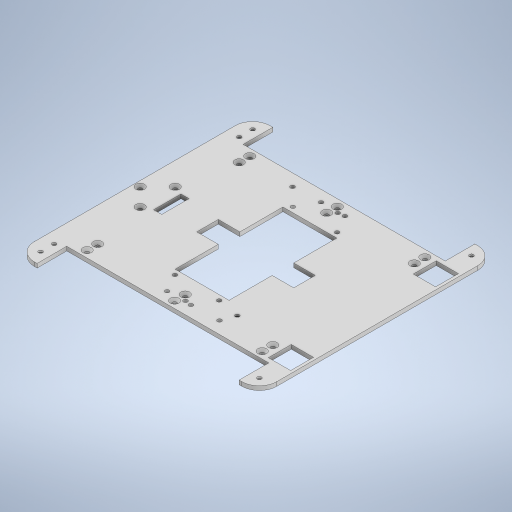
# Autodesk Inventor part: base
Saved by Autodesk Inventor 2023 (Build 270158000, 158)
## iProperties
Created: 2026-02-09
Part Number: base
Material: Типовые
Document SubType Name: Modeling
Designer: garin
Density: 1 g/cm^3
Appearance: По умолчанию
Author: garin
Autodesk Inventor part; units mm, degrees
ref_plane "YZ Plane" through (0, 0, 0) normal (1, 0, 0) x (0, 1, 0)
ref_plane "XZ Plane" through (0, 0, 0) normal (0, 1, 0) x (-1, 0, 0)
ref_plane "XY Plane" through (0, 0, 0) normal (0, 0, 1) x (1, 0, 0)
sketch "Эскиз1" plane through (0, 0, 0) normal (0, 1, 0) x (-1, 0, 0)
  line L0 (-77, -87.5) -> (77, -87.5)
  line L1 (90, -74.5) -> (90, 74.5)
  line L2 (77, 87.5) -> (-77, 87.5)
  line L3 (-90, 74.5) -> (-90, -74.5)
  line L4 (90, 0) -> (-90, 0) construction
  line L5 (0, -87.5) -> (0, 87.5) construction
  arc A0 (90, 74.5) -> (77, 87.5) centre (77, 74.5) ccw
  arc A1 (77, -87.5) -> (90, -74.5) centre (77, -74.5) ccw
  arc A2 (-90, -74.5) -> (-77, -87.5) centre (-77, -74.5) ccw
  arc A3 (-77, 87.5) -> (-90, 74.5) centre (-77, 74.5) ccw
  line L6 (75, 83.5) -> (-75, 83.5)
  line L7 (-75, 83.5) -> (-75, 65.5)
  line L8 (-75, 65.5) -> (75, 65.5)
  line L9 (75, 65.5) -> (75, 83.5)
  line L10 (0, 87.5) -> (0, -87.5) construction
  line L11 (75, -83.5) -> (-75, -83.5)
  line L12 (-75, -83.5) -> (-75, -65.5)
  line L13 (-75, -65.5) -> (75, -65.5)
  line L14 (75, -65.5) -> (75, -83.5)
  line L15 (90, 49.8397) -> (90, 20.3597)
  line L16 (0, 65.5) -> (42, 65.5)
  line L17 (90, -32.9125) -> (90, 38.6688)
  line L18 (68, 60) -> (-12, 60)
  line L19 (-12, 60) -> (-12, -60)
  line L20 (-12, -60) -> (68, -60)
  line L21 (68, -60) -> (68, 60)
  line L22 (60, 60) -> (57.2, 60)
  line L23 (60, 57.2) -> (60, 60)
  circle A4 centre (65.2, 57.2) radius 1.5
  line L24 (20, 60) -> (20, -60) construction
  circle A5 centre (65.2, -57.2) radius 1.5
  circle A6 centre (-9.2, 57.2) radius 1.5
  circle A7 centre (-9.2, -57.2) radius 1.5
  line L25 (-20, 0) -> (-25, 0) construction
  line L26 (-25, 0) -> (-81, 0) construction
  line L27 (-13, 42.5) -> (-69, 42.5)
  line L28 (-69, 42.5) -> (-69, -42.5)
  line L29 (-69, -42.5) -> (-13, -42.5)
  line L30 (-13, -42.5) -> (-13, 42.5)
  line L31 (-25, 42.5) -> (-28.7, 42.5)
  line L32 (-25, 38.8) -> (-25, 42.5)
  circle A8 centre (-16.7, 38.8) radius 1.5
  line L33 (-53, 42.5) -> (-53, -42.5) construction
  line L34 (-25, 0) -> (-81, 0) construction
  line L35 (-16.7, 38.8) -> (-16.7, -19.2) construction
  circle A9 centre (-16.7, -19.2) radius 1.5
  circle A10 centre (-65.3, 38.8) radius 1.5
  circle A11 centre (-65.3, -19.2) radius 1.5
  line L36 (90, 60.5) -> (90, 65.5)
  circle A12 centre (65, 60.3847) radius 1.5
  circle A13 centre (65, 52.5) radius 1.5
  line L37 (32.5, 60.3847) -> (32.5, -60) construction
  circle A14 centre (0, 60.3847) radius 1.5
  circle A15 centre (0, 52.5) radius 1.5
  circle A16 centre (-65, 60.3847) radius 1.5
  circle A17 centre (-65, 52.5) radius 1.5
  circle A18 centre (65, -60.3847) radius 1.5
  circle A19 centre (65, -52.5) radius 1.5
  circle A20 centre (0, -60.3847) radius 1.5
  circle A21 centre (0, -52.5) radius 1.5
  circle A22 centre (-65, -60.3847) radius 1.5
  circle A23 centre (-65, -52.5) radius 1.5
  circle A24 centre (86, 0) radius 1.5
  line L38 (86, 0) -> (104.385, 0) construction
  circle A25 centre (72.9998, -13.0002) radius 1.5
  circle A26 centre (72.9998, 12.9998) radius 1.5
  line L39 (90, -19.2) -> (75, -19.2)
  line L40 (75, -19.2) -> (75, 22.1472)
  line L41 (75, 22.1472) -> (90, 22.1472)
  line L42 (90, 22.1472) -> (90, -19.2)
  line L43 (-90, 8.1057) -> (-90, 0)
  line L44 (0, 0) -> (-12, 0)
  line L45 (-12, 5.1924) -> (-12, 5.1924)
  line L46 (75, 78.692) -> (75, 65.5)
  circle A27 centre (81.192, 78.692) radius 1.5
  circle A28 centre (81.192, -78.692) radius 1.5
  circle A29 centre (81.192, 68.692) radius 1.5
  circle A30 centre (81.192, -68.692) radius 1.5
  line L47 (66.2, 9.8) -> (66.2, -10.5)
  line L48 (66.2, -10.5) -> (60.2, -10.5)
  line L49 (60.2, -10.5) -> (60.2, 9.8)
  line L50 (60.2, 9.8) -> (66.2, 9.8)
  circle A31 centre (-81.192, -78.692) radius 1.5
  circle A32 centre (-81.192, 78.692) radius 1.5
  line L51 (0, 0) -> (-71.5, 0) construction
  line L52 (-71.5, 0) -> (-71.5, 45.306) construction
  line L53 (-71.5, 45.306) -> (0, 45.306) construction
  line L54 (0, 45.306) -> (0, 0) construction
  line L55 (-71.5, 45.306) -> (-88, 45.306)
  line L56 (-88, 45.306) -> (-88, 62.3062)
  line L57 (-88, 62.3062) -> (-71.5, 62.3062)
  line L58 (-71.5, 62.3062) -> (-71.5, 45.306)
  line L59 (-71.5, -45.306) -> (-88, -45.306)
  line L60 (-88, -45.306) -> (-88, -62.3062)
  line L61 (-88, -62.3062) -> (-71.5, -62.3062)
  line L62 (-71.5, -62.3062) -> (-71.5, -45.306)
  line L63 (20, -40) -> (-20, -40)
  line L64 (-20, -40) -> (-20, 40)
  line L65 (-20, 40) -> (20, 40)
  line L66 (20, 40) -> (20, -40)
  line L67 (20, 0) -> (-20, 0) construction
  line L68 (0, -40) -> (0, 40) construction
  line L69 (0, 65.5) -> (-4.2, 65.5) construction
  line L70 (-4.2, 65.5) -> (-4.2, 56.5) construction
  line L71 (-4.2, 56.5) -> (0, 56.5) construction
  line L72 (0, 56.5) -> (0, 65.5) construction
  circle A33 centre (-4.2, 56.5) radius 1.5
  line L73 (0, 65.5) -> (-29.4, 65.5) construction
  line L74 (-29.4, 65.5) -> (-29.4, 56.5) construction
  line L75 (-29.4, 56.5) -> (0, 56.5) construction
  line L76 (0, 56.5) -> (0, 65.5) construction
  circle A34 centre (-29.4, 56.5) radius 1.5
  circle A35 centre (-4.2, -56.5) radius 1.5
  circle A36 centre (29.4, -56.5) radius 1.5
  line L77 (0, 60.3847) -> (8.833, 60.3847)
  line L78 (8.833, 60.3847) -> (8.833, 57.162)
  line L79 (8.833, 57.162) -> (0, 57.162)
  line L80 (0, 57.162) -> (0, 60.3847)
  circle A37 centre (8.833, 57.162) radius 1.5
  circle A38 centre (-8.833, 57.162) radius 1.5
  circle A39 centre (8.833, -57.162) radius 1.5
  circle A40 centre (-8.833, -57.162) radius 1.5
  line L81 (-20, 0) -> (-20, -8)
  line L82 (-20, -8) -> (-36, -8)
  line L83 (-36, -8) -> (-36, 8)
  line L84 (-36, 8) -> (-20, 8)
  line L85 (-20, 8) -> (-20, -8)
  line L86 (20, -8) -> (36, -8)
  line L87 (36, -8) -> (36, 8)
  line L88 (36, 8) -> (20, 8)
  line L89 (20, 8) -> (20, -8)
  line L90 (0, 0) -> (16.43, 0) construction
  line L91 (16.43, 0) -> (16.43, 43.8) construction
  line L92 (16.43, 43.8) -> (0, 43.8) construction
  line L93 (0, 43.8) -> (0, 0) construction
  circle A41 centre (16.43, 43.8) radius 1.5
  circle A42 centre (-16.43, 43.8) radius 1.5
  circle A43 centre (16.43, -43.8) radius 1.5
  circle A44 centre (-16.43, -43.8) radius 1.5
  line L94 (0, 0) -> (-32.9, 0) construction
  line L95 (-32.9, 0) -> (-32.9, 46.85) construction
  line L96 (-32.9, 46.85) -> (0, 46.85) construction
  line L97 (0, 46.85) -> (0, 0) construction
  circle A45 centre (-32.9, 46.85) radius 1.5
  line L98 (0, -83.5) -> (3, -83.5)
  line L99 (3, -83.5) -> (-3, -83.5)
  line L100 (-3, -83.5) -> (-3, -65.5)
  line L101 (-3, -65.5) -> (3, -65.5)
  line L102 (3, -65.5) -> (3, -83.5)
  line L103 (-3, 83.5) -> (-3, 65.5)
  line L104 (3, 65.5) -> (3, 83.5)
  line L105 (75, 83.5) -> (75, 87.5)
  line L106 (-75, 83.5) -> (-75, 87.5)
  line L107 (75, -83.5) -> (75, -87.5)
  line L108 (-75, -83.5) -> (-75, -87.5)
  point P0 (90, 87.5)
  point P1 (90, -87.5)
  point P2 (-90, 87.5)
  point P3 (-77, -74.5)
  point P4 (60, 0)
  point P5 (75, 0)
  point P6 (60, 0)
  point P7 (-60, 0)
  point P8 (-4, 0)
  point P9 (-5, 0)
  point P10 (-15, 0)
  point P11 (-70, 0)
  point P12 (-14, 0)
  point P13 (-28.7, -19.2)
  point P14 (-17.7, -19.2)
  point P15 (-13, 0)
  point P16 (-14, 0)
  point P17 (-17.6, 40)
  point P18 (-15.8, 40)
  dimension "d0" = 180
  dimension "d1" = 175
  dimension "d2" = 13
  dimension "d7" = 150
  dimension "d8" = 18
  dimension "d13" = 80
  dimension "d14" = 120
  dimension "d21" = 56
  dimension "d22" = 85
  dimension "d25" = 3
  dimension "d26" = 58
  dimension "d27" = 3
  dimension "d30" = 3
  dimension "d32" = 3
  dimension "d33" = 32.5
  dimension "d54" = 3
  dimension "d58" = 3
  dimension "d59" = 3
  dimension "d60" = 15
  dimension "d62" = 12
  dimension "d68" = 3
  dimension "d70" = 3
  dimension "d72" = 20.3
  dimension "d73" = 6
  dimension "d76" = 3
  dimension "d77" = 71.5
  dimension "d78" = 45.306
  dimension "d79" = 40
  dimension "d80" = 80
  dimension "d81" = 4.2
  dimension "d82" = 9
  dimension "d83" = 3
  dimension "d84" = 29.4
  dimension "d85" = 9
  dimension "d86" = 3
  dimension "d87" = 3
  dimension "d88" = 8
  dimension "d89" = 16
  dimension "d90" = 16
  dimension "d91" = 16.43
  dimension "d92" = 43.8
  dimension "d93" = 3
  dimension "d94" = 3
  dimension "d104" = 3
  dimension "d105" = 6
  constraints: 218 end point, 46 centre point, 42 symmetric about line, 31 parallel, 26 point on line, 21 perpendicular, 19 horizontal, 13 midpoint, 11 coincident, 8 point on circle, 8 tangent, 3 equal radius, 2 vertical, 20 other
  measures "d0" distance of point (-90, 87.5) point (90, 87.5)
  measures "d1" distance of point (90, 87.5) point (90, -87.5)
  measures "d2" radius of A0
  measures "d7" distance of L8.end L7.end
  measures "d8" distance of L7.end L6.end
  measures "d13" distance of L20.end L19.end
  measures "d14" distance of L19.end L18.end
  measures "d21" distance of L29.start L29.end
  measures "d22" distance of L28.end L28.start
  measures "d25" diameter of A8
  measures "d26" distance of L35.start L35.end
  measures "d27" diameter of A9
  measures "d30" diameter of A12
  measures "d32" diameter of A13
  measures "d33" distance of A12.centre L37.start
  measures "d54" diameter of A24
  measures "d58" diameter of A25
  measures "d59" diameter of A26
  measures "d60" distance of L40.end L41.end
  measures "d62" distance of L44.start L44.end
  measures "d68" diameter of A27
  measures "d70" diameter of A29
  measures "d72" distance of L47.start L47.end
  measures "d73" distance of L47.end L48.end
  measures "d76" diameter of A31
  measures "d77" distance of L52.end L53.end
  measures "d78" distance of L51.end L52.end
  measures "d79" distance of L64.end L65.end
  measures "d80" distance of L63.end L64.end
  measures "d81" distance of L71.end L70.end
  measures "d82" distance of L70.end L69.end
  measures "d83" diameter of A33
  measures "d84" distance of L75.end L74.end
  measures "d85" distance of L74.end L73.end
  measures "d86" diameter of A34
  measures "d87" diameter of A37
  measures "d88" distance of L67.end L81.end
  measures "d89" distance of L83.end L84.end
  measures "d90" distance of L82.end L83.end
  measures "d91" distance of L92.end L91.end
  measures "d92" distance of L91.end L90.end
  measures "d93" diameter of A41
  measures "d94" diameter of A45
  measures "d104" distance of L98.start L98.end
  measures "d105" distance of L100.end L101.end
sketch "Эскиз2" plane through (0, 0, 0) normal (0, 1, 0) x (-1, 0, 0)
  line L0 (77, 87.5) -> (-77, 87.5)
  line L1 (-90, 74.5) -> (-90, -74.5)
  line L2 (-77, -87.5) -> (77, -87.5)
  line L3 (90, -74.5) -> (90, 74.5)
  line L4 (90, 0) -> (-90, 0) construction
  line L5 (0, 87.5) -> (0, -87.5) construction
  arc A0 (90, 74.5) -> (77, 87.5) centre (77, 74.5) ccw
  arc A1 (-77, 87.5) -> (-90, 74.5) centre (-77, 74.5) ccw
  arc A2 (-90, -74.5) -> (-77, -87.5) centre (-77, -74.5) ccw
  arc A3 (77, -87.5) -> (90, -74.5) centre (77, -74.5) ccw
  line L6 (150, -150) -> (-150, -150)
  line L7 (-150, -150) -> (-150, 150)
  line L8 (-150, 150) -> (150, 150)
  line L9 (150, 150) -> (150, -150)
  line L10 (150, 0) -> (-150, 0) construction
  line L11 (0, -150) -> (0, 150) construction
  circle A4 centre (0, 0) radius 150
  line L12 (75, -74.5) -> (75, -83.5)
  line L13 (75, -83.5) -> (-75, -83.5)
  line L14 (-75, -83.5) -> (-75, -65.5)
  line L15 (-75, -65.5) -> (75, -65.5)
  line L16 (75, -65.5) -> (75, -83.5)
  line L17 (75, 74.5) -> (75, 83.5)
  line L18 (75, 83.5) -> (-75, 83.5)
  line L19 (-75, 83.5) -> (-75, 65.5)
  line L20 (-75, 65.5) -> (75, 65.5)
  line L21 (75, 65.5) -> (75, 83.5)
  line L22 (0, -65.5) -> (42, -65.5)
  line L23 (42, -65.5) -> (77, -65.5)
  line L24 (77, -65.5) -> (77, -82.3082)
  line L25 (77, -82.3082) -> (42, -82.3082)
  line L26 (77, -65.5) -> (7, -65.5)
  line L27 (7, -65.5) -> (7, -82.3082)
  line L28 (7, -82.3082) -> (77, -82.3082)
  line L29 (77, -82.3082) -> (77, -65.5)
  line L30 (-42, -65.5) -> (-77, -65.5)
  line L31 (-77, -65.5) -> (-77, -82.3082)
  line L32 (-7, -65.5) -> (-7, -82.3082)
  line L33 (-7, -82.3082) -> (-77, -82.3082)
  line L34 (42, -65.5) -> (29.5, -65.5)
  line L35 (29.5, -10.5) -> (54.5, -10.5)
  line L36 (54.5, -10.5) -> (54.5, -65.5)
  line L37 (54.5, -65.5) -> (29.5, -65.5)
  line L38 (29.5, -65.5) -> (29.5, -10.5)
  line L39 (29.5, 10.5) -> (54.5, 10.5)
  line L40 (54.5, 10.5) -> (54.5, 65.5)
  line L41 (29.5, 65.5) -> (29.5, 10.5)
  line L42 (-29.5, -10.5) -> (-54.5, -10.5)
  line L43 (-54.5, -10.5) -> (-54.5, -65.5)
  line L44 (-29.5, -65.5) -> (-29.5, -10.5)
  line L45 (-29.5, 65.5) -> (-29.5, 10.5)
  line L46 (-29.5, 10.5) -> (-54.5, 10.5)
  line L47 (-54.5, 10.5) -> (-54.5, 65.5)
  point P0 (0, 0)
  point P1 (-90, -87.5)
  point P2 (-90, 87.5)
  point P3 (90, -87.5)
  point P4 (-80.411, -84.4848)
  point P5 (77, 74.5)
  point P6 (-7, -73.9041)
  point P7 (7, -73.9041)
  dimension "d34" = 180
  dimension "d35" = 175
  dimension "d36" = 13
  dimension "d37" = 300
  dimension "d38" = 300
  dimension "d41" = 150
  dimension "d42" = 18
  dimension "d44" = 35
  dimension "d45" = 70
  dimension "d46" = 14
  dimension "d47" = 84
  dimension "d50" = 25
  constraints: 96 end point, 24 symmetric about line, 13 midpoint, 11 parallel, 9 point on line, 9 tangent, 8 point on circle, 7 horizontal, 6 perpendicular, 5 centre point, 3 equal radius, 2 coincident
  measures "d34" distance of point (90, -87.5) point (-90, -87.5)
  measures "d35" distance of point (-90, -87.5) point (-90, 87.5)
  measures "d36" radius of A0
  measures "d37" distance of L7.end L8.end
  measures "d38" distance of L6.end L7.end
  measures "d41" distance of L14.end L15.end
  measures "d42" distance of L13.end L14.end
  measures "d44" distance of L24.end L25.end
  measures "d45" distance of L28.end L27.end
  measures "d46" distance of point (-7, -73.904) point (7, -73.904)
  measures "d47" distance of L30.start L34.start
  measures "d50" distance of L36.end L37.end
extrude "Выдавливание1" add sketch "Эскиз1" along normal blind 3 contours A2 L3 A3 L2 L106 L7 L8 L9 L105 A0 L1 L41 L40 L39 A1 L0 L107 L14 L13 L12 L108 | L39 L40 L41 L1 | L18 A12 L21 L20 A18 A20 L19 L63 L66 L86 L87 L88 L65 A14 L80 L79 A37 L78 | L78 A37 L79 L80 A14 L18 | L18 A14 L77 L78 | L65 A8 L64 L84 L83 L82 L63 L30 L29 A44 L28 L27 A42 | L65 A8 | A4 | A5 | A38 A6 | A40 A7 | A10 | A11 picked at (-16.908, 40.0547) picked at (-10.5675, 57.2211) picked at (-10.5675, -57.2211)
chamfer "Фаска3" distance 1.7 angle 45 22 edges at (-63.5, 3, 52.5) (-63.5, 3, 60.3847) (1.5, 3, 52.5) (1.5, 3, 60.3847) (66.5, 3, 52.5) (66.5, 3, 60.3847) (66.5, 3, -60.3847) (66.5, 3, -52.5) (1.5, 3, -60.3847) (1.5, 3, -52.5) (-63.5, 3, -52.5) (-63.5, 3, -60.3847) (-71.4998, 3, 12.9998) (-84.5, 3, 0) (-71.4998, 3, -13.0002) (34.4, 0, 46.85) (-79.692, 0, 78.692) (-79.692, 0, 68.692) (82.692, 0, 78.692) (82.692, 0, -78.692) (-79.692, 0, -78.692) (-79.692, 0, -68.692)
